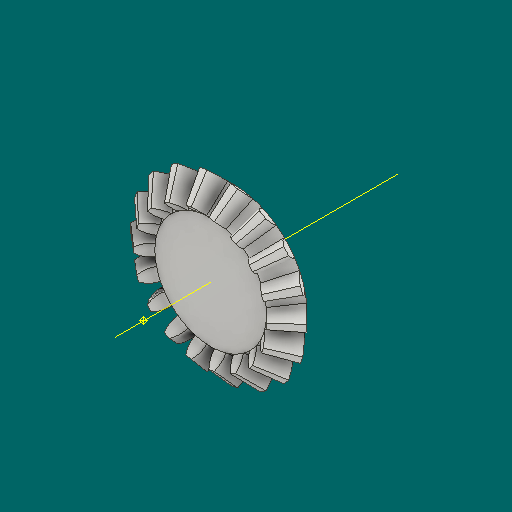
# Autodesk Inventor part: Bevel Gear1
Saved by Autodesk Inventor 2023.1 (Build 271208000, 208)
## iProperties
CustomPartVersion: 1
Created: 2022-10-09
Part Number: Bevel Gear1
Material: Steel, Mild
Document SubType Name: Modeling
Designer: zac-h
Categories: <?xml version="1.0" encoding="UTF-16"?> <MemberInstance><Categories><FamilyTemplate><FamilyTemplateParameter ValueType="xs:double" Id="1" ObjectReferenceKey="da_z" ObjectType="kUserParameterObject"/><FamilyTemplateParameter ValueType="xs:double" Id="2" ObjectReferenceKey="da_b" ObjectType="kUserParameterObject"/><FamilyTemplateParameter ValueType="xs:double" Id="3" ObjectReferenceKey="da_beta" ObjectType="kUserParameterObject"/><FamilyTemplateParameter ValueType="xs:double" Id="4" ObjectReferenceKey="da_dae" ObjectType="kUserParameterObject"/><FamilyTemplateParameter ValueType="xs:double" Id="5" ObjectReferenceKey="da_ve" ObjectType="kUserParameterObject"/><FamilyTemplateParameter ValueType="xs:double" Id="6" ObjectReferenceKey="da_omega" ObjectType="kUserParameterObject"/><FamilyTemplateParameter ValueType="xs:string" Id="7" ObjectReferenceKey="EAIAABAAAAAAHwAAAAAAAIAAAAAAAAAA" ObjectType="83914240" SubObjectId="SurfaceGeometry"/></FamilyTemplate><ParamToTemplateMap><ParamToTemplate CategoryParameter="//CategoryParameter[@InternalName='046C89C9-8512-4d59-83FE-43B91F4F132A']" TemplateParameter="1"/><ParamToTemplate CategoryParameter="//CategoryParameter[@InternalName='2552DF32-E462-4b46-AEBF-C6C7768E72AC']" TemplateParameter="2"/><ParamToTemplate CategoryParameter="//CategoryParameter[@InternalName='C9EE641D-15FC-4fae-A226-E94C4372FDD7']" TemplateParameter="3"/><ParamToTemplate><ParamToTemplate CategoryParameter="//CategoryParameter[@InternalName='00B6519A-459B-49c7-AD84-2E56D39A5744']" ConstantValue="0.000000"/></ParamToTemplate><ParamToTemplate><ParamToTemplate CategoryParameter="//CategoryParameter[@InternalName='04B31F0E-C7A6-4894-AA32-9629BEFACF47']" ConstantValue="1.000000"/></ParamToTemplate><ParamToTemplate><ParamToTemplate CategoryParameter="//CategoryParameter[@InternalName='43CBEC2E-7847-49e7-A936-2F7889FCB2D9']" ConstantValue="0.200000"/></ParamToTemplate><ParamToTemplate><ParamToTemplate CategoryParameter="//CategoryParameter[@InternalName='B1EFC894-105D-4ebd-86BF-FA20ED196853']" ConstantValue="0.266800"/></ParamToTemplate><ParamToTemplate><ParamToTemplate CategoryParameter="//CategoryParameter[@InternalName='51175063-3D10-4879-93E8-6246FE8B403D']" ConstantValue="2061532430.657340"/></ParamToTemplate><ParamToTemplate><ParamToTemplate CategoryParameter="//CategoryParameter[@InternalName='A3A52E27-4454-46a9-B0BD-C932399B70AF']" ConstantValue="0.300000"/></ParamToTemplate><ParamToTemplate CategoryParameter="//CategoryParameter[@InternalName='2A200944-5A8C-41ca-B96E-8520D2E510F1']" TemplateParameter="4"/><ParamToTemplate><ParamToTemplate CategoryParameter="//CategoryParameter[@InternalName='1A637F62-92C8-44bc-B81F-10802510B579']" ConstantValue="1.855475"/></ParamToTemplate><ParamToTemplate CategoryParameter="//CategoryParameter[@InternalName='B52DD4BE-6863-48fb-BF58-89EF6F9EC65C']" TemplateParameter="5"/><ParamToTemplate><ParamToTemplate CategoryParameter="//CategoryParameter[@InternalName='3956BFF2-84D2-457d-93C2-9B0613DEBA67']" ConstantValue="0.792577"/></ParamToTemplate><ParamToTemplate CategoryParameter="//CategoryParameter[@InternalName='739CFA02-461B-4bf8-8049-181FCAD8B28F']" TemplateParameter="6"/><ParamToTemplate><ParamToTemplate CategoryParameter="//CategoryParameter[@InternalName='A27E999F-E2CE-4481-8A2A-EBF499C4C3C5']" ConstantValue="0.000000"/></ParamToTemplate><ParamToTemplate><ParamToTemplate CategoryParameter="//CategoryParameter[@InternalName='9E1B4470-B2D3-4ff1-B813-535BB4CDF51A']" ConstantValue="3523220.976809"/></ParamToTemplate><ParamToTemplate><ParamToTemplate CategoryParameter="//CategoryParameter[@InternalName='F8452263-BFF6-458c-9FB1-07C4B99E95CD']" ConstantValue="11397033.805607"/></ParamToTemplate><ParamToTemplate><ParamToTemplate CategoryParameter="//CategoryParameter[@InternalName='3E3BB259-FD49-497f-8171-6EBC954A3479']" ConstantValue="2.000000"/></ParamToTemplate><ParamToTemplate CategoryParameter="//CategoryParameter[@InternalName='27C3BAF2-7550-4e4b-AE2C-0DB134B7D9B7']" TemplateParameter="7"/></ParamToTemplateMap><Category DisplayName="Gear" InternalName="DC85795E-93AB-48d5-8EEE-5A27447B64BD" Mnemonic="Gear"><CategoryParameter DisplayName="z" InternalName="046C89C9-8512-4d59-83FE-43B91F4F132A" Mnemonic="z"/><CategoryParameter DisplayName="b" InternalName="2552DF32-E462-4b46-AEBF-C6C7768E72AC" Mnemonic="b"/><CategoryParameter DisplayName="||b|" InternalName="C9EE641D-15FC-4fae-A226-E94C4372FDD7" Mnemonic="beta"/><CategoryParameter DisplayName="x" InternalName="00B6519A-459B-49c7-AD84-2E56D39A5744" Mnemonic="x"/><CategoryParameter DisplayName="a*" InternalName="04B31F0E-C7A6-4894-AA32-9629BEFACF47" Mnemonic="a"/><CategoryParameter DisplayName="c*" InternalName="43CBEC2E-7847-49e7-A936-2F7889FCB2D9" Mnemonic="c"/><CategoryParameter DisplayName="r|.f|*" InternalName="B1EFC894-105D-4ebd-86BF-FA20ED196853" Mnemonic="rf"/><CategoryParameter DisplayName="E" InternalName="51175063-3D10-4879-93E8-6246FE8B403D" Mnemonic="E"/><CategoryParameter DisplayName="||m|" InternalName="A3A52E27-4454-46a9-B0BD-C932399B70AF" Mnemonic="mi"/><Category DisplayName="BevelGear" InternalName="0C98F69A-0C2B-4791-B2FE-7691BB227E77" Mnemonic="BevelGear"><CategoryParameter DisplayName="d|.ae|" InternalName="2A200944-5A8C-41ca-B96E-8520D2E510F1" Mnemonic="dae"/><CategoryParameter DisplayName="d|.ai|" InternalName="1A637F62-92C8-44bc-B81F-10802510B579" Mnemonic="dai"/><CategoryParameter DisplayName="A|.e|" InternalName="B52DD4BE-6863-48fb-BF58-89EF6F9EC65C" Mnemonic="ve"/><CategoryParameter DisplayName="A|.i|" InternalName="3956BFF2-84D2-457d-93C2-9B0613DEBA67" Mnemonic="vi"/><CategoryParameter DisplayName="||S|" InternalName="739CFA02-461B-4bf8-8049-181FCAD8B28F" Mnemonic="omega"/><CategoryParameter DisplayName="x|.t|" InternalName="A27E999F-E2CE-4481-8A2A-EBF499C4C3C5" Mnemonic="xt"/><CategoryParameter DisplayName="||s||.Flim|" InternalName="9E1B4470-B2D3-4ff1-B813-535BB4CDF51A" Mnemonic="sFlim"/><CategoryParameter DisplayName="||s||.Hlim|" InternalName="F8452263-BFF6-458c-9FB1-07C4B99E95CD" Mnemonic="sHlim"/><CategoryParameter DisplayName="type" InternalName="3E3BB259-FD49-497f-8171-6EBC954A3479" Mnemonic="type"/><CategoryParameter DisplayName="PitchDiameter" InternalName="27C3BAF2-7550-4e4b-AE2C-0DB134B7D9B7" Mnemonic="IDS_PITCHDIAM"/></Category></Category></Categories></MemberInstance>
Mass: 60.9118 g
Surface Area: 34.3074 cm^2
Volume: 7.7496 cm^3
Density: 7.86 g/cm^3
Appearance: Steel
Author: zac-h
Autodesk Inventor part; units mm, degrees
ref_plane "Mesh Plane2" through (0, 0, 0) normal (0.9848078, 0.1736482, 0) x (0, 0, 1)
sketch "Teeth Body Sketch" plane through (0, 0, 0) normal (1, 0, 0) x (0, 1, 0)
  line L0 (0, 0) -> (10.352369, -12.507631) construction
  line L1 (10.352369, -12.507631) -> (12.328026, -10.531974)
  line L2 (12.328026, -10.531974) -> (0, 0) construction
  line L3 (11.43, -11.43) -> (0, 0) construction
  line L4 (7.790609, -9.412537) -> (9.277376, -7.92577)
  line L5 (10.352369, -12.507631) -> (7.790609, -9.412537)
  line L6 (12.328026, -10.531974) -> (9.277376, -7.92577)
  line L7 (0, -13.485157) -> (0, 2.247526)
  line L8 (0, -11.43) -> (12.328026, -11.43) construction
  dimension "d0" = 22.86
  dimension "d1" = 20.70474
  dimension "d2" = 24.65605
  dimension "d3" = 4
  dimension "d4" = 10.53197
  constraints: 16 end point, 4 point on line, 3 perpendicular, 2 collinear, 1 horizontal alignment, 1 vertical alignment
  measures "d0" diameter of L3.start L7
  measures "d1" diameter of L0.end L7
  measures "d2" diameter of L1.end L7
  measures "d3" distance between parallel lines of L1 L4
  measures "d4" vertical distance of L1.end L0.start
revolve "Teeth Body" add sketch "Teeth Body Sketch" angle 360 about axis through (0, 0, 0) along (0, 0, 1)
ref_plane "Tooth Plane" through (0, 11.43, -11.43) normal (0, -0.7071068, 0.7071068) x (1, 0, 0)
sketch "Start Sketch" plane through (0, 11.43, -11.43) normal (0, -0.7071068, 0.7071068) x (1, 0, 0)
  line L0 (0, -6.650226) -> (0, 16.474152)
  arc A0 (-0.748646, -1.85928) -> (-2.354705, 1.955846) centre (-5.357012, -1.553656) ccw
  arc A1 (2.354705, 1.955846) -> (0.748646, -1.85928) centre (5.357012, -1.553656) ccw
  line L1 (-0.748646, -1.85928) -> (0.748646, -1.85928)
  arc A2 (2.354705, 1.955846) -> (-2.354705, 1.955846) centre (0, -16.164461) ccw
  dimension "d7" = 4.61849
  dimension "d8" = 5.35701
  dimension "d9" = 14.6108
  dimension "d57" = 18.27266
  dimension "d58" = 14.30518
  constraints: 6 point on circle, 3 centre point, 3 symmetric about line, 2 end point, 1 coincident, 1 perpendicular, 1 other
  measures "d7" radius of A0
  measures "d8" horizontal distance of point (0, -16.164) A0.centre
  measures "d9" vertical distance of point (0, -16.164) A0.centre
  measures "d57" radius of A2
  measures "d58" distance from line of A2.centre L1
sketch "End Sketch" plane through (0, 8.50279, -8.50279) normal (0, -0.7071068, 0.7071068) x (1, 0, 0)
  line L0 (0, -4.323522) -> (0, 12.138464)
  arc A0 (-0.556918, -1.383121) -> (-1.751668, 1.454956) centre (-3.985088, -1.155767) ccw
  arc A1 (1.751668, 1.454956) -> (0.556918, -1.383121) centre (3.985088, -1.155767) ccw
  line L1 (-0.556918, -1.383121) -> (0.556918, -1.383121)
  arc A2 (1.751668, 1.454956) -> (-1.751668, 1.454956) centre (0, -12.024761) ccw
  dimension "d12" = 3.4357
  dimension "d15" = 3.98509
  dimension "d16" = 10.86899
  dimension "d59" = 13.59305
  dimension "d60" = 10.64164
  constraints: 6 point on circle, 3 centre point, 3 symmetric about line, 2 end point, 1 coincident, 1 other
  measures "d12" radius of A0
  measures "d15" horizontal distance of A0.centre point (0, -12.025)
  measures "d16" vertical distance of A0.centre point (0, -12.025)
  measures "d59" radius of A2
  measures "d60" distance from line of A2.centre L1
loft "Loft" cut profiles "Start Sketch", "End Sketch"
pattern_circular "Circular Pattern" count 18 over 360 about axis through (0, 0, 0) along (0, 0, 1) of "Loft"
ref_plane "End Plane" through (0, 8.50279, -8.50279) normal (0, -0.7071068, 0.7071068) x (1, 0, 0)
sketch3d "3D Sketch Right"
ref_plane "End Plane Right" through (-2.19352, 8.214981, -8.50279) normal (0.1824169, -0.6831721, 0.7071068) x (0.9661512, 0.2579765, 0)
sketch "End Sketch Right" plane through (-2.19352, 8.214981, -8.50279) normal (0.1824169, -0.6831721, 0.7071068) x (0.9661512, 0.2579765, 0)
  arc A0 (-0.556918, -1.383121) -> (-1.751668, 1.454956) centre (-3.985088, -1.155767) ccw
  line L0 (0, -18.112741) -> (0, 15.874732)
  arc A1 (1.751668, 1.454956) -> (0.556918, -1.383121) centre (3.985088, -1.155767) ccw
  line L1 (-0.556918, -1.383121) -> (0.556918, -1.383121)
  arc A2 (1.751668, 1.454956) -> (-1.751668, 1.454956) centre (0, -12.024761) ccw
  dimension "d70" = 3.98509
  dimension "d71" = 10.86899
  dimension "d72" = 3.4357
  dimension "d73" = 10.64164
  dimension "d74" = 13.59305
  constraints: 6 point on circle, 3 centre point, 3 symmetric about line, 2 end point, 1 coincident, 1 perpendicular, 1 other
  measures "d70" horizontal distance of A2.centre A0.centre
  measures "d71" vertical distance of point (0, -12.025) A0.centre
  measures "d72" radius of A0
  measures "d73" distance from line of point (0, -12.025) L1
  measures "d74" radius of A2
feature "Loft Right" [suppressed]
pattern_circular "Circular Pattern Right" [suppressed]
sketch3d "3D Sketch Left"
ref_plane "End Plane Left" through (2.22859, 8.214981, -8.529401) normal (-0.1849448, -0.6817395, 0.7078324) x (0.9651166, -0.2618203, 0)
sketch "End Sketch Left" plane through (2.22859, 8.214981, -8.529401) normal (-0.1849448, -0.6817395, 0.7078324) x (0.9651166, -0.2618203, 0)
  line L0 (0, -20.366351) -> (0, 18.129989)
  arc A0 (-0.556918, -1.370768) -> (-1.751668, 1.467308) centre (-3.985088, -1.143414) ccw
  arc A1 (1.751668, 1.467308) -> (0.556918, -1.370768) centre (3.985088, -1.143414) ccw
  line L1 (-0.556918, -1.370768) -> (0.556918, -1.370768)
  ellipse E0 centre (0, -5.598608) end of major axis (9.277376, -5.598608) minor radius 6.566828
  arc A2 (1.751668, 1.467308) -> (-1.751668, 1.467308) centre (0, -12.012409) ccw
  dimension "d56" = 6.56683
  dimension "d30" = 3.4357
  dimension "d31" = 3.98509
  dimension "d32" = 10.86899
  dimension "d61" = 13.59305
  dimension "d62" = 10.64164
  constraints: 6 point on circle, 3 centre point, 3 symmetric about line, 2 end point, 1 coincident, 2 other
  measures "d30" radius of A0
  measures "d31" horizontal distance of point (0, -12.012) A0.centre
  measures "d32" vertical distance of A0.centre point (0, -12.012)
  measures "d61" radius of A2
  measures "d62" distance from line of point (0, -12.012) L1
feature "Loft Left" [suppressed]
pattern_circular "Circular Pattern Left" [suppressed]
sketch "Body Sketch" plane through (0, 0, 0) normal (1, 0, 0) x (0, 1, 0)
  line L0 (0, -11.863316) -> (0, -7.483518)
  line L1 (10.352369, -12.507631) -> (7.790609, -9.412537)
  line L2 (7.790609, -9.412537) -> (0, -9.412537)
  line L3 (10.352369, -12.507631) -> (0, -12.507631)
  constraints: 4 end point, 2 perpendicular, 2 point on line
sketch "Body Sketch outline for Fix Body" plane through (0, 0, 0) normal (1, 0, 0) x (0, 1, 0)
  line L0 (0, -12.507631) -> (10.352369, -12.507631)
  line L1 (0, -9.412537) -> (0, -12.507631)
  line L2 (7.790609, -9.412537) -> (0, -9.412537)
  line L3 (10.352369, -12.507631) -> (7.790609, -9.412537)
revolve "Fix Body" add sketch "Body Sketch outline for Fix Body" angle 360 about axis through (0, 0, 0) along (0, 0, 1)
sketch "Sketch6" plane through (0, 0, 0) normal (1, 0, 0) x (0, 1, 0)
  line L0 (11.43, -11.43) -> (0, 0) projected
  line L1 (0, -12.192) -> (0, 2.032) projected
surface revolve "Pitch Diameter" sketch "Sketch6" angle 360 about axis through (0, 0, 0) along (0, 0, 1) shown no curves L0
equation "\"d0\" = da_de"
equation "\"d1\" = da_dfe"
equation "\"d2\" = da_dae"
equation "\"d3\" = da_b"
equation "\"d4\" = da_ve"
equation "\"d7\" = fd_rr"
equation "\"d8\" = fd_x"
equation "\"d9\" = fd_y"
equation "\"d57\" = 0.5 * fd_dva + 0.3 * da_he"
equation "\"d58\" = 0.5 * fd_dva - 1.12 * da_he"
equation "\"da_teethtype\" = 0"
equation "\"da_b\" = 4"
equation "\"da_de\" = 22.86"
equation "\"da_dae\" = 24.65605"
equation "\"da_dfe\" = 20.70474"
equation "\"da_le\" = 16.16446"
equation "\"da_omega\" = 90deg"
equation "\"da_beta\" = 0"
equation "\"da_delta\" = 45deg"
equation "\"da_alpha\" = 14.5deg"
equation "\"da_he\" = 2.794"
equation "\"da_ve\" = 10.53197"
equation "\"da_zv\" = 25.455844"
equation "\"fd_loft\" = da_b + 0.05 * da_he"
equation "\"fd_x\" = fd_x1 + fd_x2"
equation "\"fd_y\" = fd_y1 - fd_y2"
equation "\"fd_dd\" = fd_dva - 0.8 * da_he"
equation "\"da_dvw\" = 32.32892"
equation "\"d11\" = fd_loft"
equation "\"da_dm\" = 20.03157"
equation "\"da_x\" = 0"
equation "\"da_m\" = 1.27"
equation "\"d50\" = da_omega"
equation "\"fd_rr\" = 4.61849"
equation "\"fd_dva\" = 34.868922"
equation "\"fd_x1\" = 0.996823"
equation "\"fd_x2\" = 4.36019"
equation "\"fd_y1\" = 16.133696"
equation "\"fd_y2\" = 1.522891"
body "Solid1"
body "Srf1"
